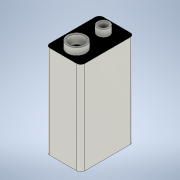
# Autodesk Inventor part: battery model
Saved by Autodesk Inventor 2020 (Build 240168000, 168)
## iProperties
Created: 2021-07-08
Part Number: battery model
Material: Generic
Document SubType Name: Modeling
Designer: legoo
Density: 1 g/cm^3
Appearance: Default
Author: legoo
Autodesk Inventor part; units mm, degrees
ref_plane "YZ Plane" through (0, 0, 0) normal (1, 0, 0) x (0, 1, 0)
ref_plane "XZ Plane" through (0, 0, 0) normal (0, 1, 0) x (-1, 0, 0)
ref_plane "XY Plane" through (0, 0, 0) normal (0, 0, 1) x (1, 0, 0)
sketch "Sketch1" plane through (0, 0, 0) normal (0, 1, 0) x (-1, 0, 0)
  line L0 (0, 0) -> (-17, 0)
  line L1 (-17, 0) -> (-17, -26)
  line L2 (-17, -26) -> (0, -26)
  line L3 (0, -26) -> (0, 0)
  dimension "d0" = 26
  dimension "d1" = 17
  constraints: 8 end point, 2 parallel, 1 horizontal, 1 perpendicular
  measures "d0" distance of L2.end L0.start
  measures "d1" distance of L1.end L2.end
extrude "Extrusion1" add sketch "Sketch1" along normal blind 45
fillet "Fillet1" radius 2 4 edges at (0, 22.5, -26) (0, 22.5, 0) (17, 22.5, -26) (17, 22.5, 0)
sketch "Sketch2" plane through (0, 45, 0) normal (0, 1, 0) x (1, 0, 0)
  circle A0 centre (8.5, 19.5) radius 2.875
  line L0 (15, 26) -> (2, 26) projected
  circle A1 centre (8.5, 6.5) radius 4.5
  line L1 (0, 24) -> (0, 2) projected
  line L2 (2, 0) -> (15, 0) projected
  point P0 (0, 0)
  dimension "d5" = 5.75
  dimension "d6" = 6.5
  dimension "d7" = 9
  dimension "d8" = 8.5
  dimension "d9" = 8.5
  dimension "d10" = 6.5
  constraints: 2 centre point
  measures "d5" diameter of A0
  measures "d6" distance from line of A0.centre L0
  measures "d7" diameter of A1
  measures "d8" distance from line of A0.centre L1
  measures "d9" distance from line of L1 A1.centre
  measures "d10" distance from line of L2 A1.centre
extrude "Extrusion2" add sketch "Sketch2" along normal blind 3.3
shell "Shell1" thickness 1 removed faces 2 at (7.7246, 48.3, -18.7113) at (10.0336, 48.3, -5.5053)
body "Solid1"
